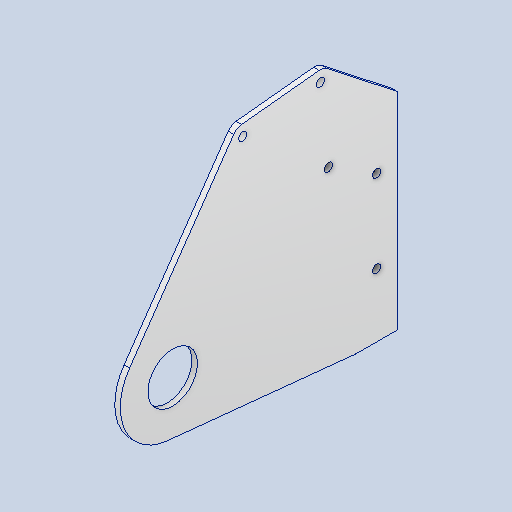
# Autodesk Inventor part: hand-grab-v5-Plate-6
Saved by Autodesk Inventor 2025.2 (Build 292293000, 293)
## iProperties
Created: 2025-05-11
Part Number: hand-grab-v5-Plate-6
Material: アルミニウム 6061
Document SubType Name: Modeling
Designer: haruy
Density: 2.7 g/cm^3
Appearance: アルミニウム - フラット
Author: haruy
Autodesk Inventor part; units mm, degrees
ref_plane "YZ Plane" through (0, 0, 0) normal (1, 0, 0) x (0, 1, 0)
ref_plane "XZ Plane" through (0, 0, 0) normal (0, 1, 0) x (-1, 0, 0)
ref_plane "XY Plane" through (0, 0, 0) normal (0, 0, 1) x (1, 0, 0)
derived "dribl-v3-Sketch-Base.ipt"
sketch "スケッチ1" plane through (400, 0, 0) normal (1, 0, 0) x (0, 1, 0)
  circle A0 centre (0, 0) radius 120 construction
  circle A1 centre (-96.5237, 35.1318) radius 6.5 projected
  line L0 (0, 0) -> (-96.5237, 35.1318) projected
  line L1 (0, 0) -> (0, 120) projected
  line L2 (246.0862, 200) -> (-251.4603, 200) projected
  circle A2 centre (-67.6203, 200) radius 6.5 projected
  line L3 (0, 0) -> (-120, 0) projected
  line L4 (248, 9.15) -> (186, 9.15) projected
  line L5 (186, 9.15) -> (186, -9.15) projected
  line L6 (186, -9.15) -> (248, -9.15) projected
  line L7 (248, -9.15) -> (248, 9.15) projected
  line L8 (186, 5.15) -> (178, 5.15) projected
  line L9 (178, 5.15) -> (178, -4.85) projected
  line L10 (178, -4.85) -> (186, -4.85) projected
  line L11 (186, -4.85) -> (186, 5.15) projected
  line L12 (178, 3.15) -> (173, 3.15) projected
  line L13 (173, 3.15) -> (173, -2.85) projected
  line L14 (173, -2.85) -> (178, -2.85) projected
  line L15 (178, -2.85) -> (178, 3.15) projected
  line L16 (173, 2.65) -> (158, 2.65) projected
  line L17 (158, 2.65) -> (158, -2.35) projected
  line L18 (158, -2.35) -> (173, -2.35) projected
  line L19 (173, -2.35) -> (173, 2.65) projected
  line L20 (186, 34.15) -> (184, 34.15) projected
  line L21 (184, 34.15) -> (184, -47.85) projected
  line L22 (184, -47.85) -> (186, -47.85) projected
  line L23 (186, -47.85) -> (186, 34.15) projected
  circle A3 centre (150, 65) radius 4 projected
  circle A4 centre (150, 65) radius 14 construction
  line L24 (186, 34.15) -> (191, 34.15) projected
  line L25 (191, 34.15) -> (191, 14.15) projected
  line L26 (191, 14.15) -> (186, 14.15) projected
  line L27 (186, 14.15) -> (186, 34.15) projected
  line L28 (184, 34.15) -> (147.5804, 61.8148) projected
  line L29 (151.3835, 68.7531) -> (191, 54.15) projected
  line L30 (191, 54.15) -> (191, 34.15) projected
  line L31 (239.3868, 130) -> (-239.3868, 130) projected
  circle A5 centre (-96.5237, 35.1318) radius 4 projected
  circle A6 centre (150, 65) radius 9 projected
  line L32 (-92.7649, 33.7637) -> (-100.2825, 36.4998) projected
  line L33 (165, 36) -> (150, 36) projected
  circle A7 centre (150, 36) radius 5 projected
  circle A8 centre (150, 36) radius 9 projected
  circle A9 centre (-98.8174, 128.095) radius 6.5 projected
  circle A10 centre (165, 36) radius 5 projected
  line L34 (150, 65) -> (165, 36) projected
  circle A11 centre (165, 36) radius 9 projected
  circle A12 centre (150, 65) radius 41.6497 projected
  line L35 (150, 65) -> (150, 36) projected
  line L36 (150, 65) -> (-96.5237, 35.1318) projected
  line L37 (-98.8174, 128.095) -> (150, 65) projected
  line L38 (150, 65) -> (150, 23.3503) projected
  circle A13 centre (150, 65) radius 32.6497 projected
  circle A14 centre (150, 32.3503) radius 9 projected
  line L39 (166.9362, 23.3503) -> (134.8586, 23.3503) projected
  line L40 (174, 3.15) -> (174, -2.85) projected
  circle A15 centre (25, 0) radius 120 projected
  line L41 (170, -52.2973) -> (211.3465, -67.3462) projected
  line L42 (211.3465, -67.3462) -> (205.1901, -84.2607) projected
  line L43 (205.1901, -84.2607) -> (163.8436, -69.2118) projected
  line L44 (163.8436, -69.2118) -> (170, -52.2973) projected
  line L45 (166.9218, -60.7546) -> (0, 0) projected
  line L46 (172.8191, -53.3234) -> (166.6627, -70.2379) projected
  line L47 (186, -47.85) -> (172.8191, -53.3234) projected
  line L48 (182.216, -56.7436) -> (176.0596, -73.6581) projected
  line L49 (186, -47.85) -> (191, -47.85) projected
  line L50 (191, -47.85) -> (191, -37.85) projected
  line L51 (191, -37.85) -> (186, -37.85) projected
  line L52 (186, -37.85) -> (186, -47.85) projected
  line L53 (191, -47.85) -> (182.216, -56.7436) projected
  circle A16 centre (221.5, -275) radius 6 construction
  line L54 (211.5, 20) -> (208.5, 20) projected
  line L55 (208.5, 20) -> (208.5, -53.7075) projected
  line L56 (208.5, -53.7075) -> (211.5, -53.7075) projected
  line L57 (211.5, -53.7075) -> (211.5, 20) projected
  line L58 (211.5, 20) -> (231.5, 20) projected
  line L59 (231.5, 20) -> (231.5, -53.7075) projected
  line L60 (231.5, -53.7075) -> (211.5, -53.7075) projected
  line L61 (211.5, -53.7075) -> (211.5, 20) projected
  line L62 (-432.3334, -230) -> (-447.3334, -230) construction
  line L63 (-447.3334, -230) -> (-447.3334, -860) construction
  line L64 (-447.3334, -860) -> (-432.3334, -860) construction
  line L65 (-432.3334, -860) -> (-432.3334, -230) construction
  line L66 (-432.3334, -250) -> (-432.3334, -230) construction
  line L67 (343, -291.5) -> (278.5, -291.5) construction
  line L68 (278.5, -291.5) -> (278.5, -334.5) construction
  line L69 (278.5, -334.5) -> (343, -334.5) construction
  line L70 (343, -334.5) -> (343, -291.5) construction
  line L71 (278.5, -291.5) -> (293.5, -291.5) construction
  line L72 (293.5, -291.5) -> (293.5, -276.5) construction
  line L73 (293.5, -276.5) -> (278.5, -276.5) construction
  line L74 (278.5, -276.5) -> (278.5, -291.5) construction
  line L75 (211.5, -53.7075) -> (231.5, -53.7075) projected
  line L76 (231.5, -53.7075) -> (231.5, -305) construction
  line L77 (231.5, -305) -> (211.5, -305) construction
  line L78 (211.5, -305) -> (211.5, -53.7075) construction
  line L79 (-432.3334, -303) -> (-447.3334, -303) projected
  line L80 (-432.3334, -303) -> (875.6666, -303) projected
  line L81 (875.6666, -303) -> (875.6666, -323) projected
  line L82 (875.6666, -323) -> (-432.3334, -323) projected
  line L83 (-432.3334, -323) -> (-432.3334, -303) projected
  line L84 (278.5, -334.5) -> (293.5, -334.5) construction
  line L85 (293.5, -334.5) -> (293.5, -349.5) construction
  line L86 (293.5, -349.5) -> (278.5, -349.5) construction
  line L87 (278.5, -349.5) -> (278.5, -334.5) construction
  line L88 (278.5, -276.5) -> (263.5, -276.5) construction
  line L89 (263.5, -276.5) -> (263.5, -359.5) construction
  line L90 (263.5, -359.5) -> (278.5, -359.5) construction
  line L91 (278.5, -359.5) -> (278.5, -276.5) construction
  circle A17 centre (221.5, -275) radius 15 construction
  line L92 (231.5, -275) -> (211.5, -275) construction
  line L93 (211.5, -275) -> (211.5, -305) construction
  line L94 (211.5, -305) -> (231.5, -305) construction
  line L95 (231.5, -305) -> (231.5, -275) construction
  line L96 (226.5, -266.3397) -> (216.5, -283.6603) construction
  line L97 (242.4808, -298.6603) -> (252.4808, -281.3397) construction
  line L98 (216.5, -283.6603) -> (242.4808, -298.6603) construction
  line L99 (-524.3334, 10.1879) -> (-524.3334, -1075.6286) construction
  line L100 (278.5, -349.5) -> (263.5, -349.5) construction
  line L101 (278.5, -276.5) -> (225.8253, -260.6372) construction
  line L102 (263.5, -349.5) -> (209.9279, -284.544) construction
  line L103 (278.5, -313) -> (263.5, -313) construction
  circle A18 centre (271, -291.5) radius 1.6 construction
  circle A19 centre (271, -334.5) radius 1.6 construction
  circle A20 centre (221.5, -275) radius 9.1 construction
  circle A21 centre (221.5, -275) radius 50 construction
  circle A22 centre (239.5, -334.8519) radius 12.5 construction
  line L104 (221.5, -275) -> (237.3114, -322.4342) construction
  line L105 (221.5, -275) -> (178.1987, -300) construction
  line L106 (221.5, -275) -> (221.5, -225) construction
  line L107 (221.5, -275) -> (254.6735, -237.5899) construction
  circle A23 centre (259.5, -334.8519) radius 4 construction
  circle A24 centre (239.5, -354.8519) radius 4 construction
  circle A25 centre (219.5, -334.8519) radius 4 construction
  line L108 (206.6714, -277.2613) -> (215.5457, -335.4549) construction
  line L109 (216.6716, -337.6803) -> (236.6716, -357.6803) construction
  line L110 (263.5, -349.5) -> (240.9941, -358.5624) construction
  circle A26 centre (259.5, -334.8519) radius 1.6 construction
  circle A27 centre (239.5, -354.8519) radius 1.6 construction
  circle A28 centre (219.5, -334.8519) radius 1.6 construction
  line L111 (-452.3334, -283) -> (-432.3334, -283) projected
  line L112 (-432.3334, -283) -> (-432.3334, -663) projected
  line L113 (-432.3334, -663) -> (-452.3334, -663) projected
  line L114 (-452.3334, -663) -> (-452.3334, -283) projected
  line L115 (-464.8334, 407.9273) -> (-464.8334, -989.4099) projected
  line L116 (1035.1666, 407.9273) -> (1035.1666, -2194.3714) projected
  line L117 (-432.3334, -643) -> (-452.3334, -643) projected
  line L118 (-432.3334, -473) -> (-464.8334, -473) projected
  line L119 (-464.8334, -88) -> (1035.1666, -88) projected
  line L120 (1035.1666, 77) -> (-464.8334, 77) projected
  line L121 (875.6666, -303) -> (1005.1666, -303) projected
  line L122 (1005.1666, -303) -> (1005.1666, -323) projected
  line L123 (1005.1666, -323) -> (875.6666, -323) projected
  line L124 (875.6666, -323) -> (875.6666, -303) projected
  line L125 (1005.1666, -303) -> (980.1666, -303) projected
  line L126 (980.1666, -303) -> (980.1666, -323) projected
  line L127 (980.1666, -323) -> (1005.1666, -323) projected
  line L128 (1005.1666, -323) -> (1005.1666, -303) projected
  circle A29 centre (964.1666, -358.18) radius 16 projected
  circle A30 centre (964.1666, -358.18) radius 7.5 projected
  line L129 (976.8707, -387.2746) -> (-428.6466, -622.1068) projected
  line L130 (-428.6466, -622.1068) -> (-425.3507, -641.8333) projected
  line L131 (-425.3507, -641.8333) -> (980.1666, -407.0011) projected
  line L132 (980.1666, -407.0011) -> (976.8707, -387.2746) projected
  line L133 (-432.3334, -643) -> (-425.3507, -641.8333) projected
  line L134 (980.1666, -323) -> (980.1666, -407.0011) projected
  line L135 (-212.3334, -323) -> (-232.3334, -323) projected
  line L136 (-232.3334, -323) -> (-232.3334, -578) projected
  line L137 (-232.3334, -578) -> (-212.3334, -578) projected
  line L138 (-212.3334, -578) -> (-212.3334, -323) projected
  line L139 (-414.8334, 0) -> (-414.8334, -960.8427) projected
  line L140 (-432.3334, -323) -> (-432.3334, -622.7228) projected
  line L141 (-232.3334, 0) -> (-232.3334, -854.7037) projected
  line L142 (-232.3334, -303) -> (-127.3334, -303) projected
  line L143 (-127.3334, -303) -> (-127.3334, -379.18) projected
  line L144 (-127.3334, -379.18) -> (-232.3334, -379.18) projected
  line L145 (-232.3334, -379.18) -> (-232.3334, -303) projected
  line L146 (-164.3334, -303) -> (-184.3334, -303) projected
  line L147 (-184.3334, -303) -> (-184.3334, -323) projected
  line L148 (-184.3334, -323) -> (-164.3334, -323) projected
  line L149 (-164.3334, -323) -> (-164.3334, -303) projected
  line L150 (985.1666, -303) -> (985.1666, -323) projected
  circle A31 centre (-222.3334, -313) radius 1.6 projected
  circle A32 centre (-202.3334, -313) radius 1.6 projected
  circle A33 centre (-222.3334, -333) radius 1.6 projected
  circle A34 centre (-222.3334, -353) radius 1.6 projected
  circle A35 centre (-139.3334, -313) radius 1.6 projected
  circle A36 centre (-149.3334, -313) radius 1.6 projected
  circle A37 centre (-143.3334, -358.18) radius 16 projected
  line L151 (948.1666, -303) -> (948.1666, -323) projected
  circle A38 centre (968.1666, -313) radius 1.5 projected
  circle A39 centre (958.1666, -313) radius 1.5 projected
  line L152 (957.1441, -390.5705) -> (960.44, -410.297) projected
  circle A40 centre (973.587, -397.9618) radius 1.5 projected
  circle A41 centre (963.7237, -399.6098) radius 1.5 projected
  line L153 (948.1666, -323) -> (948.1666, -358.18) projected
  line L154 (957.1441, -390.5705) -> (948.8361, -362.7598) projected
  circle A42 centre (-422.3334, -313) radius 1.6 projected
  circle A43 centre (-412.3334, -313) radius 1.6 projected
  circle A44 centre (-402.3334, -313) radius 1.6 projected
  circle A45 centre (-417.1354, -630.3221) radius 1.6 projected
  circle A46 centre (-407.2721, -628.6742) radius 1.6 projected
  circle A47 centre (-442.3334, -633) radius 1.6 projected
  circle A48 centre (-442.3334, -623) radius 1.6 projected
  line L155 (-452.3334, -613) -> (-432.3334, -613) projected
  line L156 (-399.0568, -617.1629) -> (-395.7609, -636.8895) projected
  line L157 (-428.6466, -622.1068) -> (-432.3334, -622.7228) projected
  line L158 (-232.3334, -193) -> (-212.3334, -193) projected
  line L159 (-212.3334, -193) -> (-212.3334, -753) projected
  line L160 (-212.3334, -753) -> (-232.3334, -753) projected
  line L161 (-232.3334, -753) -> (-232.3334, -193) projected
  line L162 (-212.3334, -443) -> (-192.3334, -443) projected
  line L163 (-192.3334, -443) -> (-192.3334, -463) projected
  line L164 (-192.3334, -463) -> (-212.3334, -463) projected
  line L165 (-212.3334, -463) -> (-212.3334, -443) projected
  line L166 (-212.3334, -593) -> (-192.3334, -593) projected
  line L167 (-192.3334, -593) -> (-192.3334, -613) projected
  line L168 (-192.3334, -613) -> (-212.3334, -613) projected
  line L169 (-212.3334, -613) -> (-212.3334, -593) projected
  line L170 (-212.3334, -638) -> (162.6666, -638) projected
  line L171 (162.6666, -638) -> (162.6666, -653) projected
  line L172 (162.6666, -653) -> (-212.3334, -653) projected
  line L173 (-212.3334, -653) -> (-212.3334, -638) projected
  line L174 (162.6666, -653) -> (177.6666, -653) projected
  line L175 (177.6666, -653) -> (177.6666, -668) projected
  line L176 (177.6666, -668) -> (162.6666, -668) projected
  line L177 (162.6666, -668) -> (162.6666, -653) projected
  line L178 (162.6666, -668) -> (147.6666, -668) projected
  line L179 (147.6666, -668) -> (147.6666, -524.7026) projected
  line L180 (147.6666, -524.7026) -> (162.6666, -524.7026) projected
  line L181 (162.6666, -524.7026) -> (162.6666, -668) projected
  circle A49 centre (155.1666, -534.7026) radius 1.6 projected
  circle A50 centre (835.5011, -421.0331) radius 1.6 projected
  circle A51 centre (855.2277, -417.7372) radius 1.6 projected
  line L182 (235.1666, 77) -> (235.1666, -1482.2484) construction
  circle A52 centre (98.7026, -266.038) radius 120 projected
  line L183 (865.1666, 77) -> (865.1666, -1796.5569) projected
  circle A53 centre (985.1666, 85) radius 120 projected
  line L184 (98.7026, -266.038) -> (38.7026, -369.961) projected
  line L185 (98.7026, -266.038) -> (98.7026, -386.038) projected
  line L186 (98.7026, -266.038) -> (-17.2085, -297.0963) projected
  line L187 (98.7026, -266.038) -> (67.6443, -150.1269) projected
  line L188 (67.6443, -150.1269) -> (-17.2085, -297.0963) projected
  line L189 (98.7026, -266.038) -> (202.6256, -326.038) projected
  line L190 (100.0335, -128.2423) -> (277.6705, -230.8011) construction
  line L191 (170.0335, -6.9988) -> (347.6705, -109.5575) construction
  line L192 (1181.4736, 111) -> (1176.4736, 111) projected
  line L193 (1176.4736, 111) -> (1176.4736, 59) projected
  line L194 (1176.4736, 59) -> (1181.4736, 59) projected
  line L195 (1181.4736, 59) -> (1181.4736, 111) projected
  line L196 (1181.4736, 95) -> (1243.4736, 95) projected
  line L197 (1243.4736, 95) -> (1243.4736, 75) projected
  line L198 (1243.4736, 75) -> (1181.4736, 75) projected
  line L199 (1181.4736, 75) -> (1181.4736, 95) projected
  line L200 (1181.4736, 90) -> (1173.4736, 90) projected
  line L201 (1173.4736, 90) -> (1173.4736, 80) projected
  line L202 (1173.4736, 80) -> (1181.4736, 80) projected
  line L203 (1181.4736, 80) -> (1181.4736, 90) projected
  line L204 (1173.4736, 87.5) -> (1153.4736, 87.5) projected
  line L205 (1153.4736, 87.5) -> (1153.4736, 82.5) projected
  line L206 (1153.4736, 82.5) -> (1173.4736, 82.5) projected
  line L207 (1173.4736, 82.5) -> (1173.4736, 87.5) projected
  line L208 (1164.4736, 87.5) -> (1128.3456, 87.5) projected
  line L209 (1128.3456, 87.5) -> (1128.3456, 82.5) projected
  line L210 (1128.3456, 82.5) -> (1164.4736, 82.5) projected
  line L211 (1164.4736, 82.5) -> (1164.4736, 87.5) projected
  line L212 (1164.4736, 87.5) -> (1164.4736, 82.5) projected
  line L213 (1161.9856, 87.5) -> (1111.9856, 87.5) projected
  line L214 (1111.9856, 87.5) -> (1111.9856, 82.5) projected
  line L215 (1111.9856, 82.5) -> (1161.9856, 82.5) projected
  line L216 (1161.9856, 82.5) -> (1161.9856, 87.5) projected
  line L217 (1136.9856, 82.5) -> (1136.9856, 87.5) projected
  line L218 (1131.9856, 121) -> (1141.9856, 121) projected
  line L219 (1141.9856, 121) -> (1141.9856, 49) projected
  line L220 (1141.9856, 49) -> (1131.9856, 49) projected
  line L221 (1131.9856, 49) -> (1131.9856, 121) projected
  line L222 (1151.9856, 82.5) -> (1121.9856, 82.5) projected
  line L223 (1121.9856, 82.5) -> (1121.9856, 72.5) projected
  line L224 (1121.9856, 72.5) -> (1151.9856, 72.5) projected
  line L225 (1151.9856, 72.5) -> (1151.9856, 82.5) projected
  line L226 (1181.4736, 111) -> (1125.6464, 111) projected
  line L227 (1125.6464, 111) -> (1125.6464, 116) projected
  line L228 (1125.6464, 116) -> (1181.4736, 116) projected
  line L229 (1181.4736, 116) -> (1181.4736, 111) projected
  line L230 (1181.4736, 59) -> (1129.1207, 59) projected
  line L231 (1129.1207, 59) -> (1129.1207, 54) projected
  line L232 (1129.1207, 54) -> (1181.4736, 54) projected
  line L233 (1181.4736, 54) -> (1181.4736, 59) projected
  line L234 (1145.2356, 111) -> (1128.7356, 111) projected
  line L235 (1128.7356, 111) -> (1128.7356, 110) projected
  line L236 (1128.7356, 110) -> (1145.2356, 110) projected
  line L237 (1145.2356, 110) -> (1145.2356, 111) projected
  line L238 (1128.7356, 59) -> (1145.2356, 59) projected
  line L239 (1145.2356, 59) -> (1145.2356, 60) projected
  line L240 (1145.2356, 60) -> (1128.7356, 60) projected
  line L241 (1128.7356, 60) -> (1128.7356, 59) projected
  line L242 (1128.4856, 110) -> (1145.4856, 110) projected
  line L243 (1145.4856, 110) -> (1145.4856, 102.5) projected
  line L244 (1145.4856, 102.5) -> (1128.4856, 102.5) projected
  line L245 (1128.4856, 102.5) -> (1128.4856, 110) projected
  line L246 (1128.4856, 60) -> (1145.4856, 60) projected
  line L247 (1145.4856, 60) -> (1145.4856, 67.5) projected
  line L248 (1145.4856, 67.5) -> (1128.4856, 67.5) projected
  line L249 (1128.4856, 67.5) -> (1128.4856, 60) projected
  line L250 (1111.9856, 85) -> (1173.4736, 85) projected
  line L251 (129.8192, -150.1425) -> (13.8924, -350.9335) construction
  line L252 (1035.1666, 327) -> (-464.8334, 327) projected
  line L253 (928.1666, -303) -> (928.1666, -323) projected
  line L254 (913.1666, -276.5) -> (898.1666, -276.5) projected
  line L255 (898.1666, -276.5) -> (898.1666, -349.5) projected
  line L256 (898.1666, -349.5) -> (913.1666, -349.5) projected
  line L257 (913.1666, -349.5) -> (913.1666, -276.5) projected
  line L258 (913.1666, -276.5) -> (928.1666, -276.5) projected
  line L259 (928.1666, -276.5) -> (928.1666, -291.5) projected
  line L260 (928.1666, -291.5) -> (913.1666, -291.5) projected
  line L261 (913.1666, -291.5) -> (913.1666, -276.5) projected
  line L262 (913.1666, -349.5) -> (928.1666, -349.5) projected
  line L263 (928.1666, -349.5) -> (928.1666, -334.5) projected
  line L264 (928.1666, -334.5) -> (913.1666, -334.5) projected
  line L265 (913.1666, -334.5) -> (913.1666, -349.5) projected
  circle A54 centre (1161.9856, -195) radius 52 projected
  line L266 (928.1666, -291.5) -> (876.1666, -291.5) projected
  line L267 (876.1666, -291.5) -> (876.1666, -301.5) projected
  line L268 (876.1666, -301.5) -> (928.1666, -301.5) projected
  line L269 (928.1666, -301.5) -> (928.1666, -291.5) projected
  line L270 (1141.9856, 116) -> (1141.9856, 54) projected
  line L271 (1151.9856, -225) -> (1151.9856, 49) projected
  line L272 (1151.9856, 49) -> (1171.9856, 49) projected
  line L273 (1171.9856, 49) -> (1171.9856, -225) projected
  line L274 (1171.9856, -225) -> (1151.9856, -225) projected
  line L275 (1141.9856, 49) -> (1124.1397, 49) projected
  line L276 (1124.1397, 49) -> (1124.1397, 47) projected
  line L277 (1124.1397, 47) -> (1141.9856, 47) projected
  line L278 (1141.9856, 47) -> (1141.9856, 49) projected
  line L279 (1151.9856, 29) -> (1171.9856, 29) projected
  circle A55 centre (405.1666, 85) radius 120 projected
  line L280 (285.1666, 327) -> (285.1666, -1249.7155) projected
  circle A56 centre (639.1666, -195) radius 52 projected
  circle A57 centre (639.1666, -195) radius 364.9055 construction
  line L281 (280.1666, 123) -> (663.4736, 123) projected
  line L282 (663.4736, 123) -> (663.4736, 47) projected
  line L283 (663.4736, 47) -> (280.1666, 47) projected
  line L284 (280.1666, 47) -> (280.1666, 123) projected
  line L285 (851.1666, -276.5) -> (1211.1666, -276.5) projected
  line L286 (1211.1666, -276.5) -> (1211.1666, -261.5) projected
  line L287 (1211.1666, -261.5) -> (851.1666, -261.5) projected
  line L288 (851.1666, -261.5) -> (851.1666, -276.5) projected
  line L289 (876.1666, -291.5) -> (861.1666, -291.5) projected
  line L290 (861.1666, -291.5) -> (861.1666, -276.5) projected
  line L291 (861.1666, -276.5) -> (876.1666, -276.5) projected
  line L292 (876.1666, -276.5) -> (876.1666, -291.5) projected
  circle A58 centre (1161.9856, -195) radius 9
  circle A59 centre (1161.9856, -195) radius 19
  circle A60 centre (1212.4447, -235.9741) radius 13
  circle A61 centre (1212.4447, -235.9741) radius 20
  circle A62 centre (1199.8373, -251.5) radius 4
  circle A63 centre (1227.9706, -248.5815) radius 4
  circle A64 centre (1225.0521, -220.4482) radius 4
  line L293 (1161.9856, -195) -> (1212.4447, -235.9741)
  line L294 (1212.4447, -235.9741) -> (1227.9706, -248.5815)
  line L295 (1172.8065, -179.3825) -> (1227.3302, -217.1603)
  line L296 (1231.9492, -248.1688) -> (1229.0308, -220.0355)
  line L297 (1231.1185, -251.0494) -> (1211.1666, -276.5)
  line L298 (1143.0819, -193.0891) -> (1136.1666, -261.5)
  line L299 (1136.1666, -261.5) -> (1136.1666, -276.5)
  circle A65 centre (1225.0521, -220.4482) radius 1.5
  circle A66 centre (1227.9706, -248.5815) radius 1.5
  circle A67 centre (1199.8373, -251.5) radius 1.5
  circle A68 centre (1189.1666, -269) radius 1.5
  circle A69 centre (1159.1666, -269) radius 1.5
  line L300 (1174.1666, -261.5) -> (1174.1666, -276.5)
  point P0 (-60, 0)
  point P1 (875.6666, -313)
  point P2 (186, 0.15)
  point P3 (186, 0)
  point P4 (1136.9856, 49)
  point P5 (851.1666, -269)
  dimension "d38" = 40
  dimension "d35" = 18
  dimension "d36" = 10
  dimension "d37" = 26
  dimension "d39" = 8
  dimension "d42" = 180
  dimension "d44" = 10
  dimension "d46" = 75
  dimension "d47" = 3
  dimension "d48" = 3
  dimension "d49" = 3
  dimension "d50" = 3
  dimension "d51" = 3
  dimension "d52" = 37
  dimension "d53" = 7.5
  dimension "d54" = 7.5
  dimension "d55" = 15
  dimension "d56" = 15
  constraints: 16 end point, 11 centre point, 7 tangent, 6 point on circle, 5 coincident, 4 point on line, 2 perpendicular, 1 collinear, 1 vertical alignment, 11 other
  measures "d35" diameter of A58
  measures "d36" radial gap between concentric circles of A58 A59
  measures "d37" diameter of A60
  measures "d39" diameter of A62
  measures "d44" distance from line of L287 A62.centre
  measures "d46" distance between parallel lines of L299 L286
  measures "d47" diameter of A65
  measures "d48" diameter of A66
  measures "d49" diameter of A67
  measures "d50" diameter of A68
  measures "d51" diameter of A69
  measures "d52" distance between parallel lines of L300 L286
  measures "d53" distance from line of A69.centre L287
  measures "d54" distance from line of A68.centre L287
  measures "d55" distance from line of A69.centre L300
  measures "d56" distance from line of A68.centre L300
extrude "押し出し2" add sketch "スケッチ1" against normal blind 2 contours L298 A54 A61 A62 A63 L297 L286 L287 | L287 L300 L285 L299 | L287 L286 L285 L300 | L298 A59 L271 L274 L273 L293 A61 A54 | A61 L293 A54 | A54 A60 L294 A63 A61 A62 | A59 L271 | A59 L273 L271 | L293 A61 A54 | A54 A61 A64 L296 A63 L294 A60 | L293 L294 A60 | A60 L294 L293 | L293 A59 L295 A54 A61 | A62 A61 A67 | A61 A67 A62 | A59 L273 L274 L271 | A63 A61 A66 | A59 L293 L273 | A54 L295 A64 A61 | A59 L273 L293 | A63 L294 A66 A61 | A64 A61 A65 | A61 A65 A64 | A63 A61 A66 L294 | A63 A61 L296 | A64 L296 A61
equation "\"d54\" = d53"
equation "\"d56\" = d55"
